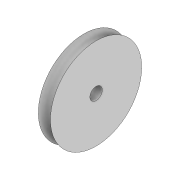
# Autodesk Inventor part: Pulley_20mm
Saved by Autodesk Inventor 2022 (Build 260153000, 153)
## iProperties
Created: 2022-07-09
Part Number: Pulley_20mm
Material: Generic
Document SubType Name: Modeling
Designer: dell
Density: 1 g/cm^3
Appearance: Default
Author: dell
Autodesk Inventor part; units mm, degrees
ref_plane "YZ Plane" through (0, 0, 0) normal (1, 0, 0) x (0, 1, 0)
ref_plane "XZ Plane" through (0, 0, 0) normal (0, 1, 0) x (-1, 0, 0)
ref_plane "XY Plane" through (0, 0, 0) normal (0, 0, 1) x (1, 0, 0)
sketch "Sketch1" plane through (0, 0, 0) normal (0, 0, 1) x (1, 0, 0)
  line L0 (-2, 0) -> (2, 0)
  line L1 (2, 0) -> (2, 15)
  line L2 (2, 15) -> (-2, 15)
  line L3 (-2, 15) -> (-2, 0)
  arc A0 (-2, 15) -> (2, 15) centre (0, 15) ccw
  line L4 (-2.8, 0) -> (2.8, 0) projected
  point P0 (0, 0)
  dimension "d0" = 4
  dimension "d1" = 2
  dimension "d2" = 15
  dimension "d3" = 2
  constraints: 8 end point, 2 parallel, 2 point on circle, 1 centre point, 1 horizontal, 1 midpoint, 1 perpendicular
  measures "d0" distance between parallel lines of L3 L1
  measures "d1" distance from line of point (0, 0) L1
  measures "d2" distance between parallel lines of L2 L0
  measures "d3" radius of A0
revolve "Revolution1" add sketch "Sketch1" angle 360 about axis through (-10, 0, 0) along (1, 0, 0) contours L3 A0 L1 L0
sketch "Sketch2" plane through (2, 0, 0) normal (1, 0, 0) x (0, 0, -1)
  circle A0 centre (0, 0) radius 2.05
  dimension "d5" = 4.1
  constraints: 1 centre point, 1 coincident
  measures "d5" diameter of A0
extrude "Extrusion1" cut sketch "Sketch2" along normal mid plane 10
equation "\"d1\" = 0.5 * d0"
body "Solid1"
